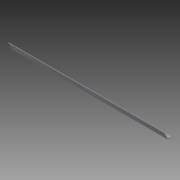
# Autodesk Inventor part: Brace Back 45
Saved by Autodesk Inventor 2015 (Build 190159000, 159)
## iProperties
Created: 2015-01-10
Part Number: Brace Back 45
Material: Generic
Document SubType Name: Modeling
Designer: Chandler Willoughby
Density: 1 g/cm^3
Appearance: Default
Author: Chandler Willoughby
Autodesk Inventor part; units mm, degrees
ref_plane "YZ Plane" through (0, 0, 0) normal (1, 0, 0) x (0, 1, 0)
ref_plane "XZ Plane" through (0, 0, 0) normal (0, 1, 0) x (-1, 0, 0)
ref_plane "XY Plane" through (0, 0, 0) normal (0, 0, 1) x (1, 0, 0)
sketch "Sketch1" plane through (0, 0, 0) normal (1, 0, 0) x (0, 1, 0)
  line L0 (0, 0) -> (25.4, 0)
  line L1 (25.4, 0) -> (25.4, -3.175)
  line L2 (25.4, -3.175) -> (3.175, -3.175)
  line L3 (3.175, -3.175) -> (3.175, -25.4)
  line L4 (3.175, -25.4) -> (0, -25.4)
  line L5 (0, -25.4) -> (0, 0)
  dimension "d0" = 25.4
  dimension "d1" = 3.175
  dimension "d2" = 22.225
  dimension "d3" = 22.225
  dimension "d4" = 3.175
  constraints: 12 end point, 4 perpendicular, 1 horizontal
  measures "d0" distance of L0.start L0.end
  measures "d1" distance of L0.end L1.end
  measures "d2" distance of L1.end L2.end
  measures "d3" distance of L2.end L3.end
  measures "d4" distance of L3.end L4.end
extrude "Extrusion1" add sketch "Sketch1" along normal blind 1022.1976
sketch "Sketch3" plane through (0, 0, 0) normal (0, 0, 1) x (1, 0, 0)
  line L0 (1022.1976, 0) -> (1022.1976, 25.4)
  line L1 (1022.1976, 25.4) -> (996.7976, 25.4)
  line L2 (996.7976, 25.4) -> (1022.1976, 0)
  line L3 (0, 25.4) -> (0, 0)
  line L4 (0, 0) -> (0, 25.4) projected
  line L5 (0, 0) -> (25.4, 0)
  line L6 (25.4, 0) -> (0, 25.4)
  dimension "d11" = 25.4
  dimension "d12" = 25.4
  dimension "d13" = 45
  constraints: 12 end point, 2 perpendicular, 1 collinear, 1 vertical
  measures "d11" distance of L0.end L1.end
  measures "d12" distance of L3.end L5.end
  measures "d13" angle of L6 L5
extrude "Extrusion3" cut sketch "Sketch3" against normal blind 1022.1976
body "Solid1"
